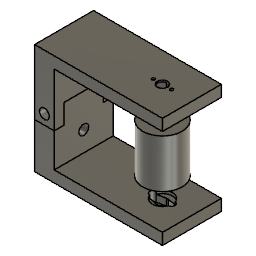
motor_stand_central_piece (Autodesk Fusion 360 design; units mm, degrees)
Autodesk Fusion 360 part; units mm, degrees
sketch "Sketch1" plane through (0, 0, 0) normal (0, 0, 1) x (1, 0, 0)
  line L0 (0, -15) -> (65, -15)
  line L1 (65, -15) -> (65, 15)
  line L2 (65, 15) -> (0, 15)
  line L3 (0, 15) -> (0, -15)
  line L4 (54.62, 0) -> (45.38, 0) construction
  line L5 (45.058, -1.7201) -> (49.5216, -2.5556)
  circle A0 centre (50, 0) radius 2.6
  circle A1 centre (54.62, 0) radius 0.8
  circle A2 centre (54.62, 0) radius 1.75
  line L6 (50.4784, -2.5556) -> (54.942, -1.7201)
  line L7 (49.5216, 2.5556) -> (45.058, 1.7201)
  line L8 (50.4784, 2.5556) -> (54.942, 1.7201)
  circle A3 centre (45.38, 0) radius 0.8
  circle A4 centre (45.38, 0) radius 1.75
  line L9 (54.62, 0) -> (65, 0) construction
  line L10 (10, -15) -> (10, 15)
  point P0 (50, 0)
  point P1 (50, 0)
  dimension "d1" = 30
  dimension "d5" = 5.2
  dimension "d6" = 9.24
  dimension "d7" = 3.5
  dimension "d8" = 1.6
  dimension "d11" = 15
  dimension "d12" = 10
  dimension "d122" = 55
  constraint horizontal L0
  constraint vertical L1
  constraint horizontal L2
  constraint vertical L3
  constraint midpoint origin L3
  constraint coincident P1 P0
  constraint midpoint P1 L4
  constraint horizontal L4
  constraint coincident L4.start A1.centre
  constraint coincident L4.end A3.centre
  constraint concentric A1 A2
  constraint concentric A3 A4
  constraint equal A2 A4
  constraint equal A1 A3
  constraint coincident L7.start A0
  constraint coincident L7.end A4
  constraint coincident L5.start A4
  constraint coincident L5.end A0
  constraint coincident L6.start A0
  constraint coincident L6.end A2
  constraint parallel L6 L7
  constraint coincident L8.start A0
  constraint coincident L8.end A2
  constraint tangent A2 L8
  constraint tangent A2 L6
  constraint tangent A0 L6
  constraint tangent A0 L8
  constraint tangent A0 L7
  constraint tangent L5 A4
  constraint tangent L5 A0
  constraint midpoint L1 L9.end
  constraint horizontal L9
  constraint coincident L0 L10.start
  constraint coincident L2 L10.end
  constraint perpendicular L2 L10
  measures "d1" distance of L0.start L2.end
  measures "d5" diameter of A0
  measures "d6" distance of L4.end L4.start
  measures "d7" diameter of A2
  measures "d8" diameter of A1
  measures "d11" distance of L1 P1
  measures "d12" distance of L3 L10
  measures "d122" distance of L1 L10
extrude "Extrude1" add sketch "Sketch1" along normal blind 0.8 contours L5 A0 L7 A4 | A4 | A0 A2 L6 L8 | A2 makes body 1 at (53.8101, 1.2278, 0.8) makes body 2 at (46.1899, -1.2278, 0)
extrude "Extrude2" add sketch "Sketch1" along normal blind 5.8 contours L0 L1 L2 L10 bodies 1 2
sketch "Sketch2" plane through (0, 0, 5.8) normal (0, 0, 1) x (-1, 0, 0)
  arc A0 (-50.4784, -2.5556) -> (-49.5216, -2.5556) centre (-50, 0) ccw
  line L0 (-50.4784, -2.5556) -> (-54.942, -1.7201)
  arc A1 (-54.942, 1.7201) -> (-54.942, -1.7201) centre (-54.62, 0) ccw
  line L1 (-54.942, 1.7201) -> (-50.4784, 2.5556)
  arc A2 (-49.5216, 2.5556) -> (-50.4784, 2.5556) centre (-50, 0) ccw
  line L2 (-49.5216, 2.5556) -> (-45.058, 1.7201)
  arc A3 (-45.058, -1.7201) -> (-45.058, 1.7201) centre (-45.38, 0) ccw
  line L3 (-45.058, -1.7201) -> (-49.5216, -2.5556)
  line L4 (-65, 15) -> (-65, -15)
  line L5 (-65, -15) -> (-10, -15)
  line L6 (-10, -15) -> (-10, 15)
  line L7 (-10, 15) -> (-65, 15)
  circle A4 centre (-50, 0) radius 5.1
  dimension "d17" = 10.2
  constraint concentric A0 A4
  measures "d17" diameter of A4
extrude "Extrude3" cut sketch "Sketch2" against normal blind 1.5 contours A0 L0 L3 A4 | L1 A2 L2 A4 bodies 1
ref_plane "WorkPlane1" through (0, 0, 56) normal (0, 0, 1) x (1, 0, 0)
sketch "Sketch5" plane through (0, 0, 56) normal (0, 0, 1) x (1, 0, 0)
  line L0 (65, -15) -> (65, 15)
  line L1 (65, 15) -> (0, 15)
  line L2 (0, -15) -> (65, -15)
  line L3 (0, 15) -> (0, -15)
  line L4 (10, -15) -> (10, 15)
  line L5 (50.4784, -2.5556) -> (54.942, -1.7201)
  line L6 (54.62, 0) -> (65, 0)
  line L7 (54.62, 0) -> (45.38, 0)
  circle A0 centre (50, 0) radius 2.6
  circle A1 centre (54.62, 0) radius 1.75
  circle A2 centre (54.62, 0) radius 0.8
  line L8 (50.4784, 2.5556) -> (54.942, 1.7201)
  line L9 (49.5216, 2.5556) -> (45.058, 1.7201)
  line L10 (45.058, -1.7201) -> (49.5216, -2.5556)
  circle A3 centre (45.38, 0) radius 1.75
  circle A4 centre (45.38, 0) radius 0.8
extrude "Extrude7" add sketch "Sketch5" against normal blind 0.8 separate body contours L5 L7 A0 A1 | L6 L7 A1 A2 | L7 A0 L10 A3 | L7 A0 A1 L8 | L6 L7 A1 A2 | L7 A0 L9 A3 | A3 makes body 3 at (46.1899, -1.2278, 56) makes body 4 at (53.8101, 1.2278, 56)
extrude "Extrude8" add sketch "Sketch5" against normal blind 5.8 contours L0 L1 L2 L4 bodies 3 4
sketch "Sketch7" plane through (0, 0, 50.2) normal (0, 0, -1) x (1, 0, 0)
  arc A0 (49.5216, -2.5556) -> (50.4784, -2.5556) centre (50, 0) ccw
  line L0 (49.5216, -2.5556) -> (45.058, -1.7201)
  arc A1 (45.058, 1.7201) -> (45.058, -1.7201) centre (45.38, 0) ccw
  line L1 (45.058, 1.7201) -> (49.5216, 2.5556)
  arc A2 (50.4784, 2.5556) -> (49.5216, 2.5556) centre (50, 0) ccw
  line L2 (50.4784, 2.5556) -> (54.942, 1.7201)
  arc A3 (54.942, -1.7201) -> (54.942, 1.7201) centre (54.62, 0) ccw
  line L3 (54.942, -1.7201) -> (50.4784, -2.5556)
  line L4 (65, -15) -> (65, 15)
  line L5 (65, 15) -> (10, 15)
  line L6 (10, 15) -> (10, -15)
  line L7 (10, -15) -> (65, -15)
  circle A4 centre (50, 0) radius 5.1
extrude "Extrude9" cut sketch "Sketch7" against normal blind 1.5 contours A0 L0 L3 A4 | L1 A2 L2 A4 bodies 3
copy_body "Body->Comp1" bodies 1 removing the originals makes body 5 in component "Bottom Stand"
copy_body "Body->Comp2" bodies 3 removing the originals makes body 6 in component "Top Stand"
sketch "Sketch12" plane through (10, 0, 0) normal (-1, 0, 0) x (0, -1, 0)
  line L0 (-15, 0) -> (15, 0)
  line L1 (15, 0) -> (15, 5.8)
  line L2 (15, 5.8) -> (-15, 5.8)
  line L3 (-15, 5.8) -> (-15, 0)
  line L4 (-15, 0) -> (-15, 23)
  line L5 (-15, 23) -> (-10, 23)
  line L6 (-10, 23) -> (-10, 33)
  line L7 (-10, 33) -> (10, 33)
  line L8 (10, 33) -> (10, 23)
  line L9 (10, 23) -> (15, 23)
  line L10 (15, 23) -> (15, 0)
  line L11 (-15, 0) -> (15, 0)
  line L12 (15, 0) -> (15, 5.8)
  line L13 (15, 5.8) -> (-15, 5.8)
  line L14 (-15, 5.8) -> (-15, 0)
  line L15 (-15, 56) -> (-15, 23)
  line L16 (15, 23) -> (15, 56)
  line L17 (15, 56) -> (-15, 56)
  line L18 (15, 56) -> (-15, 56)
  line L19 (-15, 56) -> (-15, 50.2)
  line L20 (-15, 50.2) -> (15, 50.2)
  line L21 (15, 50.2) -> (15, 56)
  line L22 (10, 28) -> (-10, 28) construction
  line L23 (10, 28) -> (10, 50.2) construction
  line L24 (10, 28) -> (10, 5.8) construction
  dimension "d86" = 10
  dimension "d87" = 5
  constraint coincident L0.start L3.end
  constraint perpendicular L0 L4
  constraint perpendicular L3 L5
  constraint perpendicular L5 L6
  constraint perpendicular L6 L7
  constraint perpendicular L7 L8
  constraint perpendicular L8 L9
  constraint coincident L0.end L1.start
  constraint perpendicular L9 L10
  constraint equal L5 L9
  constraint perpendicular L9 L16
  constraint parallel L9 L17
  constraint coincident L16.end L17.start
  constraint midpoint L8 L22.start
  constraint midpoint L6 L22.end
  constraint perpendicular L6 L22
  constraint coincident L20 L23.end
  constraint perpendicular L20 L23
  constraint coincident L2 L24.end
  constraint perpendicular L2 L24
  constraint equal L23 L24
  constraint coincident L15.start L17.end
  measures "d86" distance of L5.end L6.end
  measures "d87" distance of L4.end L5.end
extrude "Extrude1'" add sketch "Sketch12" along normal blind 10 contours L0 L1 L2 L3 L4 L10 L11 L12 L13 L14 | L2 L4 L5 L6 L7 L8 L9 L10 L13 bodies 5 in component "Bottom Stand"
extrude "Extrude1''" add sketch "Sketch12" along normal blind 10 contours L5 L6 L7 L8 L9 L15 L16 L20 | L15 L16 L17 L18 L19 L20 L21 bodies 6 in component "Top Stand"
ref_plane "WorkPlane2" through (0, 0, 15.8) normal (0, 0, 1) x (1, 0, 0)
sketch "Sketch14" plane through (0, 0, 15.8) normal (0, 0, 1) x (1, 0, 0)
  circle A0 centre (50, 0) radius 2.6 construction
  circle A1 centre (50, 0) radius 10
  circle A2 centre (50, 0) radius 5.1
  dimension "d102" = 20
  dimension "d103" = 10.2
  constraint concentric A0 A1
  constraint concentric A0 A2
  measures "d102" diameter of A1
  measures "d103" diameter of A2
extrude "Extrude14" add sketch "Sketch14" along normal blind 24.5 separate body contours A1 | A2 makes body 7
extrude "Extrude15" cut sketch "Sketch14" along normal blind 1.5 contours A2 bodies 7
sketch "Sketch15" plane through (0, 0, 40.3) normal (0, 0, 1) x (-1, 0, 0)
  circle A0 centre (-50, 0) radius 10
  circle A1 centre (-50, 0) radius 5.1
extrude "Extrude16" cut sketch "Sketch15" against normal blind 1.5 contours A1 bodies 7
sketch "Sketch16" plane through (0, -15, 0) normal (0, -1, 0) x (1, 0, 0)
  line L0 (0, 0) -> (65, 0)
  line L1 (65, 0) -> (65, 5.8)
  line L2 (65, 5.8) -> (10, 5.8)
  line L3 (10, 5.8) -> (10, 23)
  line L4 (10, 23) -> (0, 23)
  line L5 (0, 23) -> (0, 0)
  circle A0 centre (5, 28) radius 2.5
  line L6 (5, 28) -> (5, 0) construction
  dimension "d110" = 5
  dimension "d113" = 28
  dimension "d114" = 5
  constraint coincident A0.centre L6.start
  constraint perpendicular L4 L6
  constraint coincident L0 L6.end
  measures "d110" diameter of A0
  measures "d113" distance of A0.centre L6.end
  measures "d114" distance of L0.start L6.end
extrude "Extrude2'" cut sketch "Sketch16" against normal blind 30 contours A0 bodies 5 in component "Bottom Stand"
extrude "Extrude2''" cut sketch "Sketch16" against normal blind 30 contours A0 bodies 6 in component "Top Stand"
sketch "Sketch17" plane through (0, 0, 0) normal (1, 0, 0) x (0, 1, 0)
  circle A0 centre (0, 16) radius 2.5
  circle A1 centre (0, 40) radius 2.5
  line L0 (15, 23) -> (15, 0)
  line L1 (15, 0) -> (-15, 0)
  line L2 (-15, 0) -> (-15, 23)
  line L3 (-15, 23) -> (-10, 23)
  line L4 (-10, 23) -> (-10, 33)
  line L5 (-10, 33) -> (10, 33)
  line L6 (10, 33) -> (10, 23)
  line L7 (10, 23) -> (15, 23)
  line L8 (-15, 23) -> (-15, 56)
  line L9 (-15, 56) -> (15, 56)
  line L10 (15, 56) -> (15, 23)
  line L11 (15, 23) -> (10, 23)
  line L12 (10, 23) -> (10, 33)
  line L13 (10, 33) -> (-10, 33)
  line L14 (-10, 33) -> (-10, 23)
  line L15 (-10, 23) -> (-15, 23)
  line L16 (0, 0) -> (0, 16) construction
  line L17 (0, 40) -> (0, 56) construction
  dimension "d119" = 5
  dimension "d120" = 24
  constraint equal A0 A1
  constraint coincident L16.start origin
  constraint coincident A0.centre L16.end
  constraint perpendicular L1 L16
  constraint coincident A1.centre L17.start
  constraint midpoint L9 L17.end
  constraint perpendicular L9 L17
  constraint equal L16 L17
  measures "d119" diameter of A0
  measures "d120" distance of A0.centre A1.centre
extrude "Extrude3'" cut sketch "Sketch17" along normal blind 10 contours A0 | A1 bodies 5 in component "Bottom Stand"
extrude "Extrude3''" cut sketch "Sketch17" along normal blind 10 contours A0 | A1 bodies 6 in component "Top Stand"
component "Bottom Stand" placed x (1, 0, 0) y (0, 1, 0) z (0, 0, 1) at (0, 0, 0)
component "Top Stand" placed x (1, 0, 0) y (0, 1, 0) z (0, 0, 1) at (0, 0, 0)
equation "d15 = PlateThickness"
equation "d31 = Separation"
equation "PlateThickness = 5.8 mm"
equation "d35 = -PlateThickness"
equation "Separation = 56 mm" comment "original: 56"
equation "d104 = Separation - 31.5 mm"
equation "d113 = Separation / 2"
equation "Length = 55 mm" comment "original: 55"
equation "d122 = Length"
named bodies: "Bottom Stand", "Top Stand", "Middle Piece"
